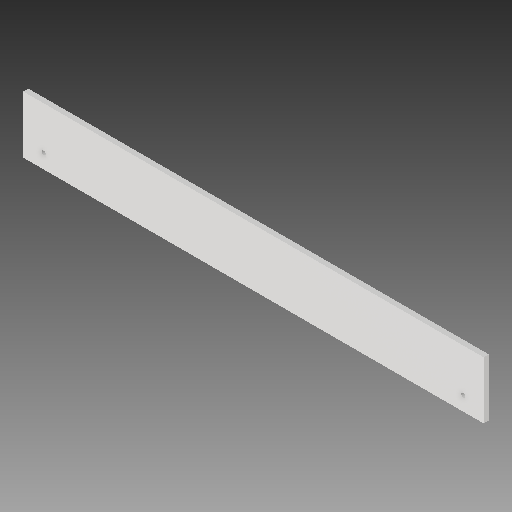
# Autodesk Inventor part: 7x56.25 Gyp
Saved by Autodesk Inventor 2017 (Build 210142000, 142)
## iProperties
Created: 2017-05-25
Part Number: 7x56.25 Gyp
Material: Generic
Document SubType Name: Modeling
Designer: cas7
Density: 1 g/cm^3
Appearance: Default
Mass: 4028.73 g
Surface Area: 5598.32 cm^2
Volume: 4028.73 cm^3
Author: cas7
Autodesk Inventor part; units mm, degrees
ref_plane "YZ Plane" through (0, 0, 0) normal (1, 0, 0) x (0, 1, 0)
ref_plane "XZ Plane" through (0, 0, 0) normal (0, 1, 0) x (-1, 0, 0)
ref_plane "XY Plane" through (0, 0, 0) normal (0, 0, 1) x (1, 0, 0)
sketch "Sketch1" plane through (0, 0, 0) normal (0, 0, 1) x (1, 0, 0)
  line L0 (0, 0) -> (1428.75, 0)
  line L1 (1428.75, 0) -> (1428.75, 177.8)
  line L2 (1428.75, 177.8) -> (0, 177.8)
  line L3 (0, 177.8) -> (0, 0)
  dimension "d0" = 1428.75
  dimension "d1" = 177.8
  constraints: 8 end point, 2 parallel, 1 horizontal, 1 perpendicular
  measures "d0" distance of L2.end L1.end
  measures "d1" distance of L1.end L0.end
extrude "Extrusion1" add sketch "Sketch1" along normal blind 15.875
sketch "Sketch2" plane through (0, 0, 0) normal (0, 0, -1) x (-1, 0, 0)
  line L0 (0, 0) -> (-63.5, 0)
  line L1 (-63.5, 0) -> (-63.5, 44.45)
  line L2 (-63.5, 44.45) -> (0, 44.45)
  line L3 (0, 44.45) -> (0, 0)
  line L4 (-1428.75, 0) -> (-1365.25, 0)
  line L5 (-1365.25, 0) -> (-1365.25, 44.45)
  line L6 (-1365.25, 44.45) -> (-1428.75, 44.45)
  line L7 (-1428.75, 44.45) -> (-1428.75, 0)
  dimension "d4" = 63.5
  dimension "d5" = 44.45
  dimension "d6" = 63.5
  dimension "d7" = 44.45
  constraints: 16 end point, 4 parallel, 2 coincident, 2 horizontal, 2 perpendicular
  measures "d4" distance of L1.end L2.end
  measures "d5" distance of L0.end L1.end
  measures "d6" distance of L6.end L5.end
  measures "d7" distance of L5.end L4.end
hole "Hole1" at (63.5, 44.45, 0) at (1365.25, 44.45, 0) at (63.5, 44.45, 0) direction (0, 0, 1) diameter 12.7 end through all
body "Solid1"
